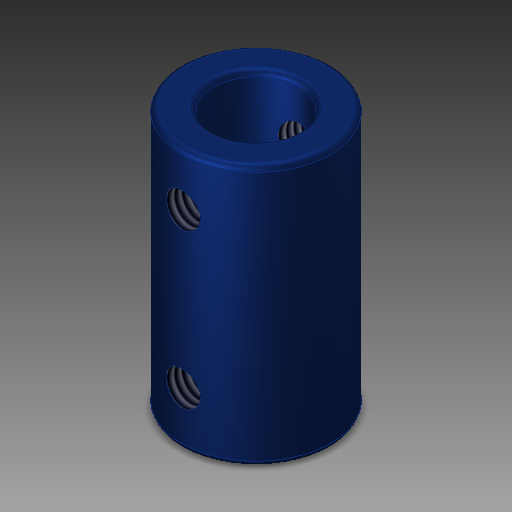
# Autodesk Inventor part: Rigid_Coupler
Saved by Autodesk Inventor 2017.3 (Build 213256000, 256)
## iProperties
Created: 2018-09-14
Part Number: Rigid_Coupler
Material: Aluminum 6061
Document SubType Name: Modeling
Designer: Ax
Density: 2.7 g/cm^3
Appearance: Anodized - Blue
Author: Ax
Autodesk Inventor part; units mm, degrees
ref_plane "YZ Plane" through (0, 0, 0) normal (1, 0, 0) x (0, 1, 0)
ref_plane "XZ Plane" through (0, 0, 0) normal (0, 1, 0) x (-1, 0, 0)
sketch "Sketch1" plane through (0, 0, 0) normal (0, 1, 0) x (-1, 0, 0)
  circle A0 centre (0, 0) radius 7
  dimension "d0" = 14
  constraints: 1 centre point, 1 coincident
  measures "d0" diameter of A0
extrude "Extrusion1" add sketch "Sketch1" along normal blind 24.5
sketch "Sketch2" plane through (0, 24.5, 0) normal (0, 1, 0) x (1, 0, 0)
  circle A0 centre (0, 0) radius 4
  dimension "d3" = 8
  constraints: 1 centre point, 1 coincident
  measures "d3" diameter of A0
extrude "Extrusion2" cut sketch "Sketch2" against normal blind 12.25
sketch "Sketch3" plane through (0, 0, 0) normal (0, -1, 0) x (1, 0, 0)
  circle A0 centre (0, 0) radius 2.5
  dimension "d6" = 5
  constraints: 1 centre point, 1 coincident
  measures "d6" diameter of A0
extrude "Extrusion3" cut sketch "Sketch3" against normal blind 12.25
fillet "Fillet1" radius 0.5 4 edges at (7, 24.5, 0) (7, 0, 0) (-4, 24.5, 0) (-2.5, 0, 0)
ref_plane "Work Plane4" through (0, 0, 7) normal (0, 0, 1) x (1, 0, 0)
sketch "Sketch8" plane through (0, 0, 7) normal (0, 0, 1) x (1, 0, 0)
  line L0 (0, 0) -> (0, 24.5) construction
  circle A0 centre (0, 5) radius 1.5
  circle A1 centre (0, 19.5) radius 1.5
  line L1 (-6.5, 24.5) -> (6.5, 24.5) projected
  dimension "d33" = 3
  dimension "d34" = 5
  dimension "d38" = 5
  constraints: 2 centre point, 2 end point, 2 point on line, 1 equal radius, 1 midpoint, 1 vertical
  measures "d33" diameter of A0
  measures "d34" distance of L0.start A0.centre
  measures "d38" distance of L0.end A1.centre
hole "Hole3" at (0, 5, 7) at (0, 19.5, 7) direction (0, 0, -1) diameter 3.242 end through all thread size "M4x0.7" class "6H" standard "ISO Metric profile"
body "Solid1"
